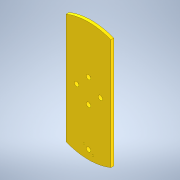
# Autodesk Inventor part: z roto base
Saved by Autodesk Inventor 2020 (Build 240168000, 168)
## iProperties
Created: 2021-01-01
Part Number: z roto base
Material: Steel, Mild
Document SubType Name: Modeling
Designer: Vikki
Density: 7.85 g/cm^3
Appearance: Glossy - Gold
Mass: 78.3619 g
Surface Area: 105.793 cm^2
Volume: 9.98241 cm^3
Author: Vikki
Autodesk Inventor part; units mm, degrees
ref_plane "YZ Plane" through (0, 0, 0) normal (1, 0, 0) x (0, 1, 0)
ref_plane "XZ Plane" through (0, 0, 0) normal (0, 1, 0) x (-1, 0, 0)
ref_plane "XY Plane" through (0, 0, 0) normal (0, 0, 1) x (1, 0, 0)
sketch "Sketch1" plane through (0, 0, 0) normal (0, 0, 1) x (1, 0, 0)
  circle A0 centre (0, 0) radius 40
  circle A1 centre (0, -8) radius 1.5
  circle A2 centre (8, 0) radius 1.5
  circle A3 centre (0, 8) radius 1.5
  circle A4 centre (-8, 0) radius 1.5
  circle A5 centre (0, -34) radius 1.5
  circle A6 centre (-3.0155, -32.086) radius 0.5 projected
  circle A7 centre (2.9845, -36.086) radius 0.5 projected
  line L0 (-15, -37.081) -> (-15, 37.081)
  line L1 (15, -37.081) -> (15, 37.081)
  dimension "d0" = 80
  dimension "d1" = 8
  dimension "d2" = 3
  dimension "d5" = 360
  dimension "d9" = 3
  dimension "d10" = 34
  dimension "d11" = 15
  dimension "d12" = 15
  constraints: 6 centre point, 4 end point, 4 point on circle, 2 vertical alignment, 1 coincident, 1 parallel, 1 vertical, 9 other
  measures "d0" diameter of A0
  measures "d1" distance of point (0, 0) A1.centre
  measures "d2" diameter of A1
  measures "d9" diameter of A5
  measures "d10" distance of point (0, 0) A5.centre
  measures "d11" distance from line of L1 point (0, 0)
  measures "d12" distance from line of point (0, 0) L0
extrude "Extrusion1" add sketch "Sketch1" along normal blind 2 contours L1 A0 L0
equation "\"d12\" = d11"
body "Solid1"
